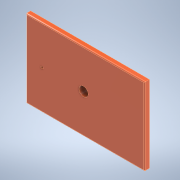
# Autodesk Inventor part: Lid
Saved by Autodesk Inventor 2022.2 (Build 262287010, 287A)
## iProperties
Created: 2022-03-17
Part Number: Lid
Material: Genérico
Document SubType Name: Modeling
Designer: mabel
Density: 1 g/cm^3
Appearance: Suave - Naranja claro
Author: mabel
Autodesk Inventor part; units mm, degrees
ref_plane "YZ Plane" through (0, 0, 0) normal (1, 0, 0) x (0, 1, 0)
ref_plane "XZ Plane" through (0, 0, 0) normal (0, 1, 0) x (-1, 0, 0)
ref_plane "XY Plane" through (0, 0, 0) normal (0, 0, 1) x (1, 0, 0)
sketch "Boceto2" plane through (0, 0, 0) normal (0, 0, 1) x (1, 0, 0)
  line L0 (130, -85) -> (-130, -85)
  line L1 (-130, -85) -> (-130, 85)
  line L2 (-130, 85) -> (130, 85)
  line L3 (130, 85) -> (130, -85)
  line L4 (130, -85) -> (-130, 85) construction
  line L5 (-130, -85) -> (130, 85) construction
  point P0 (0, 0)
  dimension "d0" = 260
  dimension "d1" = 170
  constraints: 12 end point, 2 midpoint, 2 parallel, 1 horizontal, 1 perpendicular
  measures "d0" distance of L1.end L2.end
  measures "d1" distance of L0.end L1.end
extrude "Extrusión1" add sketch "Boceto2" along normal blind 10
sketch "Boceto3" plane through (0, 0, 10) normal (0, 0, 1) x (1, 0, 0)
  line L0 (-95, 0) -> (-4.19, 0) construction
  circle A0 centre (-95, 0) radius 2.5
  circle A1 centre (-4.19, 0) radius 10
  line L1 (-130, 85) -> (-130, -85) projected
  line L2 (130, -85) -> (130, 85) projected
  line L3 (-130, -85) -> (130, -85) projected
  line L4 (130, 0) -> (80, 0) construction
  line L5 (80, 0) -> (80, -23.2237) construction
  point P0 (0, 0)
  point P1 (-130, 0)
  dimension "d7" = 5
  dimension "d8" = 20
  dimension "d14" = 85
  dimension "d29" = 50
  dimension "d30" = 90.81
  dimension "d31" = 35
  dimension "d32" = 134.19
  constraints: 6 end point, 2 centre point, 2 coincident, 2 horizontal, 2 midpoint, 1 perpendicular
  measures "d7" diameter of A0
  measures "d8" diameter of A1
  measures "d14" distance from line of L3 L0.end
  measures "d29" distance of L4.start L4.end
  measures "d30" distance of A1.centre A0.centre
  measures "d31" distance from line of A0.centre L1
  measures "d32" distance from line of L2 A1.centre
extrude "Extrusión2" cut sketch "Boceto3" against normal through all
sketch "Boceto5" plane through (0, 0, 0) normal (0, 0, -1) x (-1, 0, 0)
  line L0 (-130, -85) -> (-130, 85) projected
  line L1 (130, -85) -> (-130, -85)
  line L2 (-130, -85) -> (-130, 85)
  line L3 (-130, 85) -> (130, 85)
  line L4 (130, 85) -> (130, -85)
  line L5 (130, -85) -> (-130, 85) construction
  line L6 (-130, -85) -> (130, 85) construction
  line L7 (119, 74) -> (-119, 74)
  line L8 (-119, 74) -> (-119, -74)
  line L9 (-119, -74) -> (119, -74)
  line L10 (119, -74) -> (119, 74)
  circle A0 centre (4.19, 0) radius 10 projected
  circle A1 centre (4.19, 0) radius 20
  circle A2 centre (95, 0) radius 2.5 projected
  circle A3 centre (95, 0) radius 2.5
  point P0 (0, 0)
  dimension "d23" = 11
  dimension "d24" = 40
  dimension "d25" = 5
  constraints: 20 end point, 4 parallel, 2 centre point, 2 coincident, 2 midpoint, 2 perpendicular, 1 horizontal, 1 horizontal alignment, 3 other
  measures "d23" distance between parallel lines of L3 L7
  measures "d24" diameter of A1
  measures "d25" diameter of A3
extrude "Extrusión4" add sketch "Boceto5" along normal blind 10 contours L10 L9 L8 L7 | A1
fillet "Empalme1" radius 2 1 edges at (0, -85, 10)
fillet "Empalme2" radius 2 7 edges at (0, 85, 10) (-130, -84.4142, 9.4142) (-130, -85, 4) (-130, 1, 10) (130, -84.4142, 9.4142) (130, -85, 4) (130, 1, 10)
